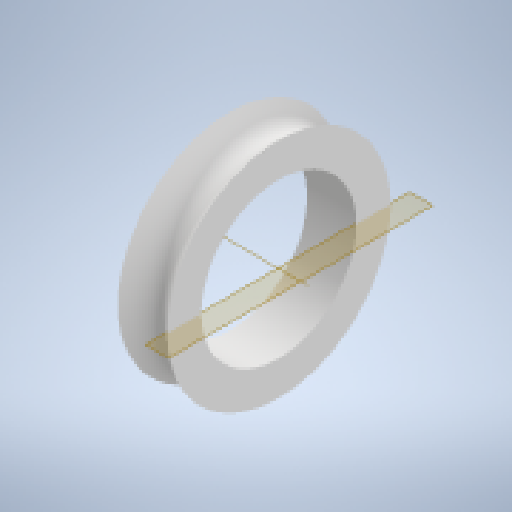
# Autodesk Inventor part: bearing cable track
Saved by Autodesk Inventor 2023 (Build 270158000, 158)
## iProperties
Created: 2023-02-17
Part Number: bearing cable track
Material: Generic
Document SubType Name: Modeling
Designer: shrey
Density: 1 g/cm^3
Appearance: Default
Author: shrey
Autodesk Inventor part; units mm, degrees
ref_plane "YZ Plane" through (0, 0, 0) normal (1, 0, 0) x (0, 1, 0)
ref_plane "XZ Plane" through (0, 0, 0) normal (0, 1, 0) x (-1, 0, 0)
ref_plane "XY Plane" through (0, 0, 0) normal (0, 0, 1) x (1, 0, 0)
ref_plane "Work Plane2" through (0, -627.55, 134.7) normal (0, 1, 0) x (1, 0, 0)
sketch "Sketch1" plane through (0, -627.55, 134.7) normal (0, 1, 0) x (1, 0, 0)
  line L0 (-3, 6.1) -> (-10, 6.1)
  line L1 (-10, 6.1) -> (-3, 6.1)
  line L2 (-3, 6.1) -> (-3, 1.2)
  line L3 (-3, 1.2) -> (-10, 1.2)
  line L4 (-10, 1.2) -> (-10, 6.1)
  spline S0 degree 2 poles (-10, 1.2) (-6.5, 5.2) (-3, 1.2) knots 0 0 0 1 1 1
  line L5 (-10, 28.2) -> (-10, 6.2) projected
  line L6 (-3, 34.4) -> (-3, 0) projected
  line L7 (2.014, 17.2) -> (-12.084, 17.2) projected
  point P0 (0, 134.7)
  point P1 (-6.5, 3.2)
  point P2 (-3, 6.1)
  dimension "d0" = 4.9
  dimension "d1" = 2
  constraints: 10 end point, 4 collinear, 2 horizontal, 2 parallel, 1 perpendicular, 3 other
  measures "d0" distance of L1.end L2.end
  measures "d1" distance from line of L3 point (-6.5, 3.2)
revolve "Revolution1" add sketch "Sketch1" angle 360 about axis through (-3, -627.55, 117.5) along (-1, 0, 0) contours L2 S0 L4 L0
body "Solid1"
